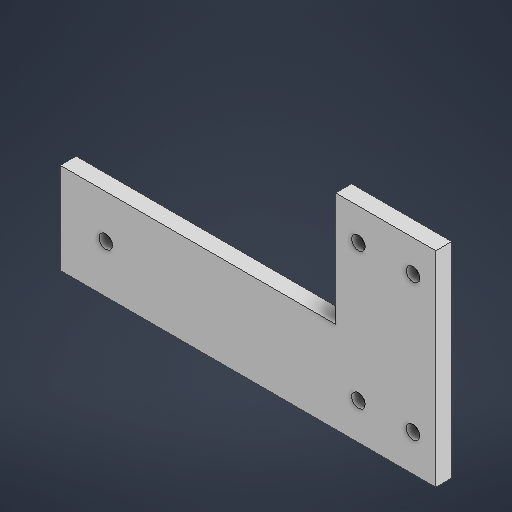
# Autodesk Inventor part: alt platform
Saved by Autodesk Inventor 2026.1 (Build 301233020, 233B)
## iProperties
Created: 2026-04-18
Part Number: alt platform
Material: Generic
Document SubType Name: Modeling
Designer: kadir
Density: 1 g/cm^3
Appearance: Default
Author: kadir
Autodesk Inventor part; units mm, degrees
ref_plane "YZ Plane" through (0, 0, 0) normal (1, 0, 0) x (0, 1, 0)
ref_plane "XZ Plane" through (0, 0, 0) normal (0, 1, 0) x (-1, 0, 0)
ref_plane "XY Plane" through (0, 0, 0) normal (0, 0, 1) x (1, 0, 0)
sketch "Sketch1" plane through (0, 0, 0) normal (0, 0, 1) x (1, 0, 0)
  line L0 (0, 0) -> (-165, 0)
  line L1 (-165, 0) -> (-165, 90)
  line L2 (-165, 90) -> (0, 90)
  line L3 (0, 90) -> (0, 0)
  line L4 (-165, 90) -> (-44, 90)
  line L5 (-44, 90) -> (-44, 40)
  line L6 (-44, 40) -> (-165, 40)
  line L7 (-165, 40) -> (-165, 90)
  dimension "d0" = 165
  dimension "d1" = 90
  dimension "d2" = 121
  dimension "d3" = 50
  constraints: 16 end point, 4 parallel, 2 horizontal, 2 perpendicular
  measures "d0" distance of L1.end L2.end
  measures "d1" distance of L0.end L1.end
  measures "d2" distance of L5.end L6.end
  measures "d3" distance of L4.end L5.end
extrude "Extrusion1" add sketch "Sketch1" along normal blind 7 contours L0 L1 L6 L5 L2 L3
sketch "Sketch2" plane through (0, 0, 7) normal (0, 0, 1) x (1, 0, 0)
  circle A0 centre (-10, 76.0401) radius 1.5
  line L0 (0, 90) -> (-44, 90) projected
  line L1 (-22, 90) -> (-22, 0)
  circle A1 centre (-34, 76.0401) radius 1.5
  circle A2 centre (-10, 16.0401) radius 1.5
  circle A3 centre (-34, 16.0401) radius 1.5
  circle A4 centre (-145, 21) radius 1.5
  line L2 (-165, 40) -> (-165, 0) projected
  line L3 (-44, 40) -> (-165, 40) projected
  line L4 (-165, 0) -> (0, 0) projected
  dimension "d6" = 3
  dimension "d7" = 24
  dimension "d8" = 3
  dimension "d9" = 60
  dimension "d10" = 3
  dimension "d11" = 20
  dimension "d15" = 21
  constraints: 5 centre point, 2 end point, 2 symmetric about line, 1 midpoint, 1 vertical, 2 other
  measures "d6" diameter of A0
  measures "d7" distance of A1.centre A0.centre
  measures "d8" diameter of A2
  measures "d9" distance of A2.centre A0.centre
  measures "d10" diameter of A4
  measures "d11" distance from line of A4.centre L2
  measures "d15" distance from line of L4 A4.centre
extrude "Extrusion2" cut sketch "Sketch2" against normal blind 10
sketch "Sketch3" plane through (0, 0, 7) normal (0, 0, 1) x (1, 0, 0)
  circle A0 centre (-10, 16.0401) radius 1.5 projected
  circle A1 centre (-10, 16.0401) radius 3
  line L0 (0, 90) -> (-44, 90) projected
  line L1 (-22, 90) -> (-22, 0)
  line L2 (-165, 0) -> (0, 0) projected
  line L3 (-22, 90) -> (68, 90) construction
  circle A2 centre (-10, 76.0401) radius 1.5 projected
  circle A3 centre (-10, 76.0401) radius 3
  circle A4 centre (-34, 16.0401) radius 3
  circle A5 centre (-34, 76.0401) radius 3
  circle A6 centre (-145, 21) radius 1.5 projected
  circle A7 centre (-145, 21) radius 3
  dimension "d16" = 6
  dimension "d17" = 90
  dimension "d18" = 6
  dimension "d19" = 6
  constraints: 5 centre point, 4 end point, 3 coincident, 2 symmetric about line, 1 horizontal, 1 midpoint, 1 perpendicular, 1 point on line, 2 other
  measures "d16" diameter of A1
  measures "d17" angle of L1 L3
  measures "d18" diameter of A3
  measures "d19" diameter of A7
extrude "Extrusion3" cut sketch "Sketch3" against normal blind 4
body "Solid1"
